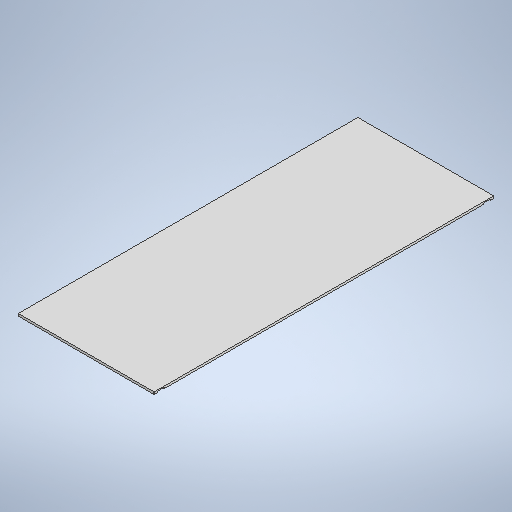
# Autodesk Inventor part: Superfície
Saved by Autodesk Inventor 2025.2 (Build 292293000, 293)
## iProperties
Created: 2025-04-02
Part Number: Superfície
Material: Genérico
Document SubType Name: Sheet Metal
Designer: kenay
Density: 1 g/cm^3
Sheet Metal Rule: Padrão_mm
Appearance: Padrão
Author: kenay
Autodesk Inventor part; units mm, degrees
ref_plane "YZ Plane" through (0, 0, 0) normal (1, 0, 0) x (0, 1, 0)
ref_plane "XZ Plane" through (0, 0, 0) normal (0, 1, 0) x (-1, 0, 0)
ref_plane "XY Plane" through (0, 0, 0) normal (0, 0, 1) x (1, 0, 0)
sketch "Esboço1" plane through (0, 0, 0) normal (0, 1, 0) x (-1, 0, 0)
  line L0 (-298, -750) -> (298, -750)
  line L1 (300, -748) -> (300, 748)
  line L2 (298, 750) -> (-298, 750)
  line L3 (-300, 748) -> (-300, -748)
  line L4 (-300, -750) -> (300, 750) construction
  line L5 (300, -750) -> (-300, 750) construction
  arc A0 (300, 748) -> (298, 750) centre (298, 748) ccw
  arc A1 (-298, 750) -> (-300, 748) centre (-298, 748) ccw
  arc A2 (298, -750) -> (300, -748) centre (298, -748) ccw
  arc A3 (-300, -748) -> (-298, -750) centre (-298, -748) ccw
  point P0 (0, 0)
  dimension "d0" = 600
  dimension "d1" = 1500
  dimension "d2" = 2
  constraints: 12 end point, 8 point on circle, 8 point on line, 8 tangent, 4 centre point, 3 equal radius, 2 midpoint, 2 parallel, 1 horizontal, 1 perpendicular
  measures "d0" distance between parallel lines of L1 L3
  measures "d1" distance between parallel lines of L0 L2
  measures "d2" radius of A0
extrude "Extrusão1" add sketch "Esboço1" along normal blind 10
sketch "Esboço3" plane through (0, 0, 0) normal (0, -1, 0) x (1, 0, 0)
  line L0 (300, -735.5) -> (-300, -735.5)
  line L1 (-300, -735.5) -> (-300, -705)
  line L2 (-300, -705) -> (300, -705)
  line L3 (300, -705) -> (300, -735.5)
  line L4 (300, -735.5) -> (-300, -705) construction
  line L5 (-300, -735.5) -> (300, -705) construction
  line L6 (-420, 0) -> (420, 0) projected
  line L7 (298, -750) -> (-298, -750) projected
  line L8 (-300, 675) -> (-300, 705)
  point P0 (0, 0)
  point P1 (0, -720.25)
  point P2 (300, -720.25)
  point P3 (-300, -720.25)
  dimension "d13" = 30.5
  dimension "d14" = 600
  dimension "d15" = 705
  dimension "d16" = 14.5
  constraints: 14 end point, 4 midpoint, 2 parallel, 1 horizontal, 1 perpendicular
  measures "d13" distance between parallel lines of L0 L2
  measures "d14" distance of point (300, -720.25) point (-300, -720.25)
  measures "d15" distance between parallel lines of L6 L2
  measures "d16" distance between parallel lines of L7 L0
extrude "Extrusão3" cut sketch "Esboço3" against normal blind 5
mirror "Espelhar1" about plane through (0, 0, 0) normal (0, 0, 1) of "Extrusão3"
equation "\"Raio_vergadura\" = Espessura"
equation "\"Largura_alívio_de_vergadura\" = Espessura"
equation "\"Profundidade_alívio_de_vergadura\" = 0.5 * Espessura"
equation "\"Tamanho_alívio_de_dobra\" = 4 * Espessura"
equation "\"Remanescente_mínimo\" = 2 * Espessura"
equation "\"Raiodetransição\" = Raio_vergadura"
equation "\"Tamanho_de_raio_de_Jacobi\" = Raio_vergadura"
equation "\"TamanhoFolga\" = Espessura"
equation "\"Espessura\" = 0.5"
